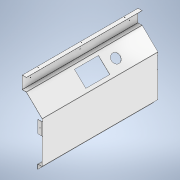
# Autodesk Inventor part: Carcaza_blanca_frontal
Saved by Autodesk Inventor 2021 (Build 250183000, 183)
## iProperties
Created: 2021-04-15
Part Number: Carcaza_blanca_frontal
Material: Acero AISI 1006 85 LC
Document SubType Name: Chapa
Designer: Admin
Density: 7.872 g/cm^3
Sheet Metal Rule: Por defecto_mm
Appearance: Blanco
Mass: 1572.03 g
Surface Area: 4365.15 cm^2
Volume: 199.698 cm^3
Author: Admin
Autodesk Inventor part; units mm, degrees
ref_plane "YZ Plane" through (0, 0, 0) normal (1, 0, 0) x (0, 1, 0)
ref_plane "XZ Plane" through (0, 0, 0) normal (0, 1, 0) x (-1, 0, 0)
ref_plane "XY Plane" through (0, 0, 0) normal (0, 0, 1) x (1, 0, 0)
sketch "Boceto1" plane through (0, 0, 0) normal (1, 0, 0) x (0, 1, 0)
  line L0 (0, 0) -> (189.4, 0)
  line L1 (189.4, 0) -> (189.4, -527.58)
  line L2 (189.4, -527.58) -> (0, -527.58)
  line L3 (0, -527.58) -> (0, 0)
  dimension "d0" = 189.4
  dimension "d1" = 527.58
  measures "d0" distance of L1.end L2.end
  measures "d1" distance of L0.end L1.end
extrude "Placa1" add sketch "Boceto1" along normal blind 0.91
sketch "Boceto2" plane through (0.91, 0.91, -527.58) normal (0, -1, 0) x (-1, 0, 0)
  line L0 (0, 527.58) -> (0, 0)
  line L1 (0, 0) -> (21.6, 0)
  line L2 (21.6, 0) -> (21.6, 527.58)
  line L3 (21.6, 527.58) -> (0, 527.58)
  constraints: 6 end point, 1 horizontal, 1 perpendicular, 1 vertical
edge flange "Pestaña1" height 21.6 angle 90 thickness 0.91 bend radius 0.91 thickness toward (0, -1, 0) relief straight relief width 0.91 relief depth 0.455 edges at (0.91, 0, -263.79) wall of the first edge with corners at (0.91, 0.91, 0) (0.91, 0.91, -527.58) (-20.69, 0.91, -527.58) (-20.69, 0.91, 0)
bend "Doblez1"
corner "Esquina1"
sketch "Boceto3" plane through (-19.78, 0.91, 0) normal (-1, 0, 0) x (0, 1, 0)
  line L0 (0, -527.58) -> (0, 0)
  line L1 (0, 0) -> (-21.6, 0)
  line L2 (-21.6, 0) -> (-21.6, -527.58)
  line L3 (-21.6, -527.58) -> (0, -527.58)
  constraints: 6 end point, 1 horizontal, 1 perpendicular, 1 vertical
edge flange "Pestaña2" height 21.6 angle 90 thickness 0.91 bend radius 0.91 thickness toward (-1, 0, 0) relief straight relief width 0.91 relief depth 0.455 edges at (-20.69, 0.91, -263.79) wall of the first edge with corners at (-19.78, 0.91, -527.58) (-19.78, 0.91, 0) (-19.78, -20.69, 0) (-19.78, -20.69, -527.58)
bend "Doblez2"
corner "Esquina2"
sketch "Boceto4" plane through (0.2791, 188.7442, 0) normal (0.6932761, 0.7206721, 0) x (0.7206721, -0.6932761, 0)
  line L0 (0, -527.58) -> (0, 0)
  line L1 (0, 0) -> (-100.563, 0)
  line L2 (-100.563, 0) -> (-100.563, -527.58)
  line L3 (-100.563, -527.58) -> (0, -527.58)
  constraints: 6 end point, 1 horizontal, 1 perpendicular, 1 vertical
edge flange "Pestaña3" height 100.563 angle 46.11 thickness 0.91 bend radius 0.91 thickness toward (0.6932761, 0.7206721, 0) relief straight relief width 0.91 relief depth 0.455 edges at (0.91, 189.4, -263.79) wall of the first edge with corners at (0.2791, 188.7442, -527.58) (0.2791, 188.7442, 0) (-72.1938, 258.4621, 0) (-72.1938, 258.4621, -527.58)
bend "Doblez3"
corner "Esquina3"
sketch "Boceto5" plane through (-71.563, 258.2079, 0) normal (0, 1, 0) x (1, 0, 0)
  line L0 (0, -527.58) -> (0, 0)
  line L1 (0, 0) -> (-20, 0)
  line L2 (-20, 0) -> (-20, -527.58)
  line L3 (-20, -527.58) -> (0, -527.58)
  constraints: 6 end point, 1 horizontal, 1 perpendicular, 1 vertical
edge flange "Pestaña4" height 20 angle 43.89 thickness 0.91 bend radius 0.91 thickness toward (0, 1, 0) relief straight relief width 0.91 relief depth 0.455 edges at (-71.563, 259.1179, -263.79) wall of the first edge with corners at (-71.563, 258.2079, -527.58) (-71.563, 258.2079, 0) (-91.563, 258.2079, 0) (-91.563, 258.2079, -527.58)
bend "Doblez4"
corner "Esquina4"
sketch "Boceto6" plane through (-90.653, 258.2079, 0) normal (-1, 0, 0) x (0, -1, 0)
  line L0 (0, -527.58) -> (0, 0)
  line L1 (0, 0) -> (-58.71, 0)
  line L2 (-58.71, 0) -> (-58.71, -527.58)
  line L3 (-58.71, -527.58) -> (0, -527.58)
  constraints: 6 end point, 1 horizontal, 1 perpendicular, 1 vertical
edge flange "Pestaña5" height 58.71 angle 90 thickness 0.91 bend radius 0.91 thickness toward (-1, 0, 0) relief straight relief width 0.91 relief depth 0.455 edges at (-91.563, 259.1179, -263.79) wall of the first edge with corners at (-90.653, 258.2079, -527.58) (-90.653, 258.2079, 0) (-90.653, 316.9179, 0) (-90.653, 316.9179, -527.58)
bend "Doblez5"
corner "Esquina5"
sketch "Boceto7" plane through (-91.563, 316.0079, -527.58) normal (0, 1, 0) x (1, 0, 0)
  line L0 (0, 527.58) -> (0, 0)
  line L1 (0, 0) -> (20, 0)
  line L2 (20, 0) -> (20, 527.58)
  line L3 (20, 527.58) -> (0, 527.58)
  constraints: 6 end point, 1 horizontal, 1 perpendicular, 1 vertical
edge flange "Pestaña6" height 20 angle 90 thickness 0.91 bend radius 0.91 thickness toward (0, 1, 0) relief straight relief width 0.91 relief depth 0.455 edges at (-91.563, 316.9179, -263.79) wall of the first edge with corners at (-91.563, 316.0079, 0) (-91.563, 316.0079, -527.58) (-71.563, 316.0079, -527.58) (-71.563, 316.0079, 0)
bend "Doblez6"
corner "Esquina6"
sketch "Boceto8" plane through (0, 1.82, 0) normal (0, 0, 1) x (1, 0, 0)
  line L0 (0.91, 186.8054) -> (0.91, 0)
  line L1 (0.91, 174.6645) -> (-19.09, 174.6645)
  line L2 (-19.09, 174.6645) -> (-19.09, 118.6317)
  line L3 (-19.09, 118.6317) -> (0.91, 118.6317)
  line L4 (0.91, 118.6317) -> (0.91, 174.6645)
  point P0 (0, -1.82)
  dimension "d63" = 20
  measures "d63" distance of L3.end L2.end
sheet face with bend "Cara2" sketch "Boceto8" thickness 0.91 toward (0, 0, -1) bend radius 0.91 relief straight relief width 0.91 relief depth 0.455
bend "Doblez7"
sketch "Boceto9" plane through (0, 1.82, -527.58) normal (0, 0, -1) x (-1, 0, 0)
  line L0 (-0.91, 174.6645) -> (-0.91, 118.6317)
  line L1 (19.09, 174.6645) -> (19.09, 118.6317)
  line L2 (-0.91, 174.6645) -> (19.09, 174.6645)
  line L3 (19.09, 174.6645) -> (19.09, 118.6317)
  line L4 (19.09, 118.6317) -> (-0.91, 118.6317)
  line L5 (-0.91, 118.6317) -> (-0.91, 174.6645)
  point P0 (0, -1.82)
sheet face with bend "Cara3" sketch "Boceto9" thickness 0.91 toward (0, 0, 1) bend radius 0.91 relief straight relief width 0.91 relief depth 0.455
bend "Doblez8"
sketch "Boceto10" plane through (0.3518, 189.937, 0) normal (0.6932761, 0.7206721, 0) x (0.7206721, -0.6932761, 0)
  line L0 (0, 527.58) -> (0, 0) projected
  line L1 (-100.3169, 0) -> (-100.3169, 527.58) projected
  line L2 (-14, 263.79) -> (-14, 318.59)
  line L3 (-14, 318.59) -> (-85.6, 318.59)
  line L4 (-85.6, 318.59) -> (-85.6, 208.99)
  line L5 (-85.6, 208.99) -> (-14, 208.99)
  line L6 (-14, 208.99) -> (-14, 263.79)
  line L7 (-49.8, 263.79) -> (-49.8, 371.79)
  circle A0 centre (-49.8, 371.79) radius 20
  point P0 (131.4253, 0)
  dimension "d75" = 54.8
  dimension "d76" = 71.6
  dimension "d77" = 109.6
  dimension "d78" = 71.6
  dimension "d81" = 108
  dimension "d82" = 40
  constraints: 12 end point, 2 perpendicular, 1 centre point, 1 coincident, 1 point on line, 1 vertical
  measures "d75" distance of L2.start L2.end
  measures "d76" distance of L2.end L3.end
  measures "d77" distance of L3.end L4.end
  measures "d78" distance of L4.end L5.end
  measures "d81" distance of L7.start L7.end
  measures "d82" diameter of A0
extrude "Extrusión1" cut sketch "Boceto10" against normal blind 10
sketch "Boceto11" plane through (0, 1.82, -527.58) normal (0, 0, -1) x (-1, 0, 0)
  line L0 (0.91, 118.6317) -> (19.09, 118.6317) construction
  line L1 (0, 174.6645) -> (-0.91, 174.6645) construction
  line L2 (19.09, 118.6317) -> (0, 174.6645) construction
  line L3 (19.09, 174.6645) -> (0.91, 174.6645) construction
  line L4 (-0.91, 118.6317) -> (0, 118.6317) construction
  line L5 (19.09, 174.6645) -> (0, 118.6317) construction
  circle A0 centre (9.545, 146.6481) radius 1.5875
  point P0 (0, -1.82)
  dimension "d83" = 3.175
  constraints: 4 end point, 1 centre point, 1 midpoint
  measures "d83" diameter of A0
extrude "Cortar1" cut sketch "Boceto11" against normal blind 0.91
sketch "Boceto12" plane through (0, 1.82, 0) normal (0, 0, 1) x (1, 0, 0)
  line L0 (-0.91, 118.6317) -> (-19.09, 118.6317) construction
  line L1 (0, 174.6645) -> (0, 118.6317) construction
  line L2 (-19.09, 118.6317) -> (0, 174.6645) construction
  line L3 (-19.09, 118.6317) -> (-19.09, 174.6645) construction
  line L4 (0, 118.6317) -> (0, 117.7217) construction
  line L5 (-19.09, 174.6645) -> (0, 118.6317) construction
  circle A0 centre (-9.545, 146.6481) radius 1.5875
  point P0 (0, -1.82)
  dimension "d86" = 3.175
  constraints: 4 end point, 1 centre point, 1 midpoint
  measures "d86" diameter of A0
extrude "Cortar2" cut sketch "Boceto12" against normal blind 0.91
sketch "Boceto13" plane through (-19.78, -20.69, 0) normal (1, 0, 0) x (0, 0, -1)
  line L0 (0, 0) -> (0, 19.78) construction
  line L1 (0, 9.89) -> (527.58, 9.89) construction
  line L2 (527.58, 19.78) -> (527.58, 0) construction
  line L3 (0, 9.89) -> (38.1, 9.89) construction
  line L4 (38.1, 9.89) -> (263.79, 9.89) construction
  line L5 (263.79, 9.89) -> (489.48, 9.89) construction
  circle A0 centre (38.1, 9.89) radius 1.5875
  circle A1 centre (263.79, 9.89) radius 1.5875
  circle A2 centre (489.48, 9.89) radius 1.5875
  point P0 (0, 20.69)
  dimension "d89" = 38.1
  dimension "d92" = 3.175
  dimension "d93" = 3.175
  dimension "d94" = 3.175
  dimension "d108" = 263.79
  dimension "d109" = 38.1
  constraints: 8 end point, 3 centre point, 3 coincident, 3 midpoint, 2 point on line
  measures "d89" distance of L1.start L3.end
  measures "d92" diameter of A0
  measures "d93" diameter of A1
  measures "d94" diameter of A2
  measures "d108" distance from line of L0 L4.end
  measures "d109" distance from line of L2 L5.end
extrude "Cortar3" cut sketch "Boceto13" against normal blind 0.91
sketch "Boceto14" plane through (-90.653, 260.0279, 0) normal (1, 0, 0) x (0, 0, -1)
  line L0 (0, 0) -> (0, 55.07) construction
  line L1 (0, 27.535) -> (527.58, 27.535) construction
  line L2 (527.58, 0) -> (527.58, 55.07) construction
  line L3 (0, 27.535) -> (38.1, 27.535) construction
  line L4 (38.1, 27.535) -> (263.79, 27.535) construction
  line L5 (263.79, 27.535) -> (489.48, 27.535) construction
  circle A0 centre (38.1, 27.535) radius 1.5875
  circle A1 centre (263.79, 27.535) radius 1.5875
  circle A2 centre (489.48, 27.535) radius 1.5875
  point P0 (0, -260.0279)
  dimension "d100" = 3.175
  dimension "d101" = 3.175
  dimension "d102" = 3.175
  dimension "d103" = 38.1
  dimension "d104" = 38.1
  dimension "d105" = 263.79
  constraints: 8 end point, 3 centre point, 3 coincident, 3 midpoint, 2 point on line
  measures "d100" diameter of A0
  measures "d101" diameter of A1
  measures "d102" diameter of A2
  measures "d103" distance from line of L0 L3.end
  measures "d104" distance from line of L2 L5.end
  measures "d105" distance from line of L0 L4.end
extrude "Cortar4" cut sketch "Boceto14" against normal blind 0.91
sketch "Boceto15" plane through (-71.563, 316.0079, -527.58) normal (0, -1, 0) x (1, 0, 0)
  circle A0 centre (-12.427, 460.725) radius 1.5875 projected
  circle A1 centre (-12.427, 263.79) radius 1.5875 projected
  circle A2 centre (-12.427, 66.855) radius 1.5875 projected
  point P0 (71.563, 527.58)
extrude "Cortar5" cut sketch "Boceto15" against normal blind 0.91
equation "\"d84\" = Grosor"
equation "\"d87\" = Grosor"
equation "\"d95\" = Grosor"
equation "\"d106\" = Grosor"
equation "\"d110\" = Grosor"
equation "\"d2\" = Grosor"
equation "\"d3\" = Anchura_desahogo_plegado"
equation "\"d4\" = Profundidad_desahogo_plegado"
equation "\"d5\" = Remanente_mínimo"
equation "\"d6\" = Radiodetransición"
equation "\"d9\" = Radio_pliegue"
equation "\"d10\" = Tamaño_destalonado"
equation "\"d11\" = TamañoSeparación"
equation "\"d12\" = Tamaño_de_radio_de_Jacobi"
equation "\"d13\" = Anchura_desahogo_plegado"
equation "\"d14\" = Profundidad_desahogo_plegado"
equation "\"d15\" = Remanente_mínimo"
equation "\"d16\" = Radiodetransición"
equation "\"d19\" = Radio_pliegue"
equation "\"d20\" = Tamaño_destalonado"
equation "\"d21\" = TamañoSeparación"
equation "\"d22\" = Tamaño_de_radio_de_Jacobi"
equation "\"d23\" = Anchura_desahogo_plegado"
equation "\"d24\" = Profundidad_desahogo_plegado"
equation "\"d25\" = Remanente_mínimo"
equation "\"d26\" = Radiodetransición"
equation "\"d29\" = Radio_pliegue"
equation "\"d30\" = Tamaño_destalonado"
equation "\"d31\" = TamañoSeparación"
equation "\"d32\" = Tamaño_de_radio_de_Jacobi"
equation "\"d33\" = Anchura_desahogo_plegado"
equation "\"d34\" = Profundidad_desahogo_plegado"
equation "\"d35\" = Remanente_mínimo"
equation "\"d36\" = Radiodetransición"
equation "\"d39\" = Radio_pliegue"
equation "\"d40\" = Tamaño_destalonado"
equation "\"d41\" = TamañoSeparación"
equation "\"d42\" = Tamaño_de_radio_de_Jacobi"
equation "\"d43\" = Anchura_desahogo_plegado"
equation "\"d44\" = Profundidad_desahogo_plegado"
equation "\"d45\" = Remanente_mínimo"
equation "\"d46\" = Radiodetransición"
equation "\"d49\" = Radio_pliegue"
equation "\"d50\" = Tamaño_destalonado"
equation "\"d51\" = TamañoSeparación"
equation "\"d52\" = Tamaño_de_radio_de_Jacobi"
equation "\"d53\" = Anchura_desahogo_plegado"
equation "\"d54\" = Profundidad_desahogo_plegado"
equation "\"d55\" = Remanente_mínimo"
equation "\"d56\" = Radiodetransición"
equation "\"d59\" = Radio_pliegue"
equation "\"d60\" = Tamaño_destalonado"
equation "\"d61\" = TamañoSeparación"
equation "\"d62\" = Tamaño_de_radio_de_Jacobi"
equation "\"d64\" = Radio_pliegue"
equation "\"d65\" = Anchura_desahogo_plegado"
equation "\"d67\" = Remanente_mínimo"
equation "\"d66\" = Profundidad_desahogo_plegado"
equation "\"d68\" = Radiodetransición"
equation "\"d69\" = Radio_pliegue"
equation "\"d70\" = Anchura_desahogo_plegado"
equation "\"d72\" = Remanente_mínimo"
equation "\"d71\" = Profundidad_desahogo_plegado"
equation "\"d73\" = Radiodetransición"
equation "\"Radio_pliegue\" = Grosor"
equation "\"Anchura_desahogo_plegado\" = Grosor"
equation "\"Profundidad_desahogo_plegado\" = 0.5 * Grosor"
equation "\"Tamaño_destalonado\" = 4 * Grosor"
equation "\"Remanente_mínimo\" = 2 * Grosor"
equation "\"Radiodetransición\" = Radio_pliegue"
equation "\"Tamaño_de_radio_de_Jacobi\" = Radio_pliegue"
equation "\"TamañoSeparación\" = Grosor"
equation "\"Grosor\" = 0.91"
